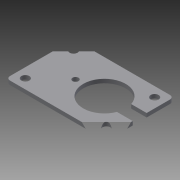
# Autodesk Inventor part: backcncld
Saved by Autodesk Inventor 2014 (Build 180170000, 170)
## iProperties
Created: 2013-06-04
Part Number: backcncld
Material: Generisch
Document SubType Name: Modeling
Designer: Felix
Density: 1 g/cm^3
Appearance: Vorgabe
Author: Felix
Autodesk Inventor part; units mm, degrees
ref_plane "YZ Plane" through (0, 0, 0) normal (1, 0, 0) x (0, 1, 0)
ref_plane "XZ Plane" through (0, 0, 0) normal (0, 1, 0) x (-1, 0, 0)
ref_plane "XY Plane" through (0, 0, 0) normal (0, 0, 1) x (1, 0, 0)
sketch "Skizze1" plane through (0, 0, 0) normal (0, 0, 1) x (1, 0, 0)
  arc A0 (26, 15.5) -> (24, 17.5) centre (24, 15.5) ccw projected
  line L0 (26, 15.5) -> (26, -15.5) projected
  arc A1 (24, -17.5) -> (26, -15.5) centre (24, -15.5) ccw projected
  line L1 (24, -17.5) -> (-24, -17.5) projected
  arc A2 (-26, -15.5) -> (-24, -17.5) centre (-24, -15.5) ccw projected
  line L2 (-26, -15.5) -> (-26, 15.5) projected
  arc A3 (-24, 17.5) -> (-26, 15.5) centre (-24, 15.5) ccw projected
  line L3 (-24, 17.5) -> (24, 17.5) projected
  circle A4 centre (-21, 12.5) radius 2.05 projected
  circle A5 centre (21, -12.5) radius 2.05 projected
  circle A6 centre (21, 12.5) radius 2.05 projected
  circle A7 centre (-21, -12.5) radius 2.05 projected
  circle A8 centre (-7.5, 0) radius 1.55 projected
  circle A9 centre (7.5, 0) radius 1.45 projected
  point P0 (0, 0)
extrude "Extrusion1" add sketch "Skizze1" along normal blind 2
sketch "Skizze2" plane through (0, 0, 2) normal (0, 0, 1) x (1, 0, 0)
  circle A0 centre (7.5, 0) radius 1.45 projected
  line L0 (14.0288, 3.3483) -> (31.2971, 3.3483)
  line L1 (31.2971, 3.3483) -> (31.2971, -3.853)
  line L2 (31.2971, -3.853) -> (14.0288, -3.853)
  line L3 (14.0288, -3.853) -> (14.0288, 3.3483)
  circle A1 centre (7.5, 0) radius 11.5
  point P0 (0, 0)
  dimension "d2" = 23
  constraints: 8 end point, 2 parallel, 1 centre point, 1 coincident, 1 horizontal, 1 perpendicular
  measures "d2" diameter of A1
extrude "Extrusion2" cut sketch "Skizze2" against normal through all
